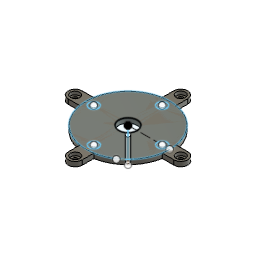
TowerLight Baseplate v13 (Autodesk Fusion 360 design; units mm, degrees)
Autodesk Fusion 360 part; units mm, degrees
sketch "Sketch1" plane through (0, 0, 0) normal (0, 1, 0) x (1, 0, 0)
  circle A0 centre (0, 0) radius 44.875
  circle A1 centre (0.067, -36.8008) radius 2.675
  line L0 (0, -44.875) -> (0, -39.475) construction
  circle A2 centre (36.8008, 0.067) radius 2.675
  circle A3 centre (-0.067, 36.8008) radius 2.675
  circle A4 centre (-36.8008, -0.067) radius 2.675
  circle A5 centre (0, 0) radius 9.85
  line L1 (0, 0) -> (31.7314, -31.7314)
  line L2 (0, 0) -> (44.875, 0) construction
  line L3 (31.7314, -31.7314, 0) -> (31.7314, -31.7314, -5) construction
  circle A6 centre (-0.067, 36.8008) radius 5
  circle A7 centre (-36.8008, -0.067) radius 5
  circle A8 centre (0.067, -36.8008) radius 5
  circle A9 centre (36.8008, 0.067) radius 5
  line L4 (31.7314, -31.7314) -> (25.4488, -38.0141) construction
  dimension "d2" = 5.35
  dimension "d3" = 5.4
  dimension "d5" = 360
  dimension "d6" = 19.7
  dimension "d16" = 45
  dimension "d19" = 5
  dimension "d27" = 10
  dimension "d29" = 360
  constraint coincident A0.centre A5.centre
  constraint coincident A0 L0.start
  constraint vertical L0
  constraint coincident A1 L0.end
  constraint horizontal L2
  constraint concentric A3 A6
  constraint tangent A0 L4
  constraint perpendicular L1 L4
  measures "d2" diameter of A1
  measures "d3" distance of L0.start L0.end
  measures "d6" diameter of A5
  measures "d16" angle of L1 L2
  measures "d19" distance of L1.end L4.start
  measures "d27" diameter of A6
extrude "Extrude1" add sketch "Sketch1" against normal blind 5 contours A0 | A1 | A2 | A3 | A4 | A6 | A7 | A8 | A9 makes body 1
extrude "Extrude2" cut sketch "Sketch1" against normal up to surface (5 mm away) contours A1 | A2 | A3 | A4 bodies 1
ref_plane "WorkPlane1" through (31.7314, -4.1197, 31.7314) normal (0.707107, 0, 0.707107) x (0.707107, 0, -0.707107)
sketch "Sketch3" plane through (31.7314, -4.1197, 31.7314) normal (0.707107, 0, 0.707107) x (0.707107, 0, -0.707107)
  line L0 (0, 4.1197) -> (0, 2.1197) construction
  line L1 (2, 4.1197) -> (-2, 4.1197)
  line L2 (-2, 4.1197) -> (-2, 2.1197)
  line L3 (2, 2.1197) -> (2, 4.1197)
  line L4 (2, 4.1197) -> (-2.0092, 0.1105) construction
  line L5 (-2, 4.1197) -> (2.0092, 0.1105) construction
  arc A0 (-2, 2.1197) -> (2, 2.1197) centre (0, 2.1197) ccw
  circle A1 through (28.6498, -0.8803, -70.9445) (24.6373, -0.8803, -68.6278) (24.6373, -0.8803, -73.2611)
  line L6 (25.9748, 4.1197, -70.9445) -> (25.9748, -0.8803, -70.9445)
  circle A2 through (-44.875, -0.8803, -44.875) (22.4375, -0.8803, -6.0121) (22.4375, -0.8803, -83.7379)
  line L7 (0, 0) -> (0, -0.8803) construction
  line L8 (0, 4.1197) -> (-8.885, 4.1197)
  point P0 (0, 4.1197)
  point P1 (0, 2.1197)
  point P2 (25.9748, 4.1197)
  dimension "d21" = 2
  dimension "d51" = 4
  constraint coincident P0 L0.start
  constraint coincident P1 L0.end
  constraint horizontal L1
  constraint perpendicular L1 L2
  constraint parallel L2 L3
  constraint coincident L4 P1
  constraint coincident L5 P1
  constraint tangent L1 A0
  constraint tangent L2 A0
  constraint perpendicular L0 L1
  constraint coincident L7.start origin
  constraint vertical L7
  constraint collinear L1 L8
  measures "d21" distance of P0 P1
  measures "d51" distance of L2 L3
ref_plane "WorkPlane2" through (0, 0, 0) normal (0, 1, 0) x (1, 0, 0)
extrude "Extrude3" cut sketch "Sketch3" against normal up to surface (44.875 mm away) bodies 1
extrude "Extrude4" cut sketch "Sketch1" along normal blind 3.5 from surface at -5 contours A6 | A7 | A8 | A9 bodies 1
sketch "Sketch4" plane through (0, -5, 0) normal (0, -1, 0) x (1, 0, 0)
  circle A0 centre (0, 0) radius 9.85
  circle A1 centre (0, 0) radius 44.875
  line L0 (-36.8008, 7.567) -> (-56.8008, 7.567)
  arc A2 (-56.8008, 7.567) -> (-56.8008, -7.433) centre (-56.8008, 0.067) ccw
  line L1 (-56.8008, -7.433) -> (-36.8008, -7.433)
  arc A3 (-36.8008, -7.433) -> (-36.8008, 7.567) centre (-36.8008, 0.067) ccw
  line L2 (-36.8008, 0.067) -> (-56.8008, 0.067) construction
  circle A4 centre (-56.8008, 0.067) radius 2.675
  circle A5 centre (-56.8008, 0.067) radius 5
  circle A6 centre (-36.8008, 0.067) radius 5
  circle A7 centre (36.8008, -0.067) radius 5
  circle A8 centre (-0.067, -36.8008) radius 5
  circle A9 centre (0.067, 36.8008) radius 5
  dimension "d32" = 15
  dimension "d33" = 5.35
  dimension "d34" = 10
  constraint tangent L0 A2
  constraint tangent A2 L1
  constraint parallel L0 L1
  constraint tangent L1 A3
  constraint tangent L0 A3
  constraint horizontal L2
  constraint concentric A2 A4
  constraint concentric A2 A5
  measures "d32" diameter of A2
  measures "d33" diameter of A4
  measures "d34" diameter of A5
copy_body "Body->Comp1" bodies 1 removing the originals makes body 2 in component "Baseplate"
extrude "Extrude5" add sketch "Sketch4" against normal up to surface (5 mm away) separate body contours A1 L0 A2 L1 makes body 3
extrude "Extrude6" add sketch "Sketch4" against normal blind 1.5 contours A5 bodies 3
pattern_circular "C-Pattern1" count 4 over 360 about axis through (0, 1.75, 0) along (0, 1, 0) of bodies 3 makes body 4 at (5.6734, -5, 51.9577) makes body 5 at (51.9577, -5, -5.6734) makes body 6 at (-5.6734, -5, -51.9577)
copy_body "CopyPasteBodies1" bodies 3 4 5 6 makes body 7 makes body 8 makes body 9 makes body 10 in component "Tabs"
move_body "Move1" bodies 7 8 9 10 to x (1, 0, 0) y (0, 1, 0) z (0, 0, 1) at (0, 0, 0) in component "Tabs"
copy_body "CopyPasteBodies2" bodies 2 makes body 11 in component "Tabs"
move_body "Move2" bodies 11 to x (1, 0, 0) y (0, 1, 0) z (0, 0, 1) at (0, 0, 0) in component "Tabs"
combine "Combine1" operation add target body 7 tool bodies 11 8 10 9 in component "Tabs"
component "Baseplate" placed x (1, 0, 0) y (0, 1, 0) z (0, 0, 1) at (0, 0, 0)
component "Tabs" placed x (1, 0, 0) y (0, 1, 0) z (0, 0, 1) at (0, 0, 0)
equation "d2 = hole_diam"
equation "d3 = hole_distance"
equation "d6 = inner_hole_diam"
equation "d9 = -height"
equation "d19 = height"
equation "d27 = counterbore_diam"
equation "d30 = counterbore_depth"
equation "d37 = -height + counterbore_depth"
equation "d41 = -height"
equation "height = 5 mm"
equation "diameter = 89.75 mm"
equation "inner_hole_diam = 19.7 mm"
equation "counterbore_diam = 10 mm"
equation "hole_diam = 5.35 mm"
equation "hole_distance = 5.4 mm"
equation "tab_length = 20 mm"
equation "counterbore_depth = 3.5 mm"
equation "wire_channel_diam = 4 mm"
equation "d51 = wire_channel_diam"
named bodies: "Baseplate", "Plate with tabs", "Baseplate only"
